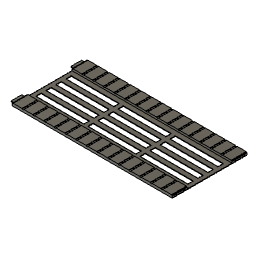
Banc de test linéaire part 2 (Autodesk Fusion 360 design; units mm, degrees)
Autodesk Fusion 360 part; units mm, degrees
sketch "Esquisse1" plane through (0, 0, 0) normal (0, 0, 1) x (1, 0, 0)
  line L0 (0, 0) -> (150, 0)
  line L1 (150, 0) -> (150, 70)
  line L2 (150, 70) -> (0, 70)
  line L3 (0, 70) -> (0, 0)
  dimension "d1" = 70
  dimension "d2" = 150
  constraint horizontal L0
  constraint vertical L1
  constraint horizontal L2
  constraint vertical L3
  constraint coincident L0.start L3.end
  measures "d1" distance of L0.start L2.end
  measures "d2" distance of L0.start L0.end
extrude "Extrusion1" add sketch "Esquisse1" along normal blind 2.5
sketch "Esquisse2" plane through (0, 0, 2.5) normal (0, 0, 1) x (-1, 0, 0)
  line L0 (0, -70) -> (0, 0)
  line L1 (0, 0) -> (-150, 0)
  line L2 (-150, 0) -> (-150, -70)
  line L3 (-150, -70) -> (0, -70)
  line L4 (0, -70) -> (-150, 0) construction
  line L5 (-150, -70) -> (0, 0) construction
  line L6 (0, -14) -> (-150, -14)
  line L7 (-150, -14) -> (-150, -56)
  line L8 (-150, -56) -> (0, -56)
  line L9 (0, -56) -> (0, -14)
  line L10 (0, -14) -> (-150, -56) construction
  line L11 (-150, -14) -> (0, -56) construction
  point P0 (-75, -35)
  dimension "d5" = 42
  dimension "d8" = 150
  constraint coincident L0.start L3.end
  constraint coincident L1.end L2.start
  constraint coincident L2.end L3.start
  constraint coincident L0.end L1.start
  constraint horizontal L6
  constraint perpendicular L6 L7
  constraint parallel L6 L8
  constraint parallel L7 L9
  constraint coincident L10 P0
  constraint coincident L11 P0
  constraint midpoint L4 P0
  measures "d5" distance of L6.end L7.end
  measures "d8" distance of L6.start L6.end
extrude "Extrusion2" cut sketch "Esquisse2" against normal blind 2 contours L0 L2 L6 L7 L8 L9
sketch "Esquisse3" plane through (0, 0, 2.5) normal (0, 0, 1) x (-1, 0, 0)
  line L0 (-150, -14) -> (0, -14)
  line L1 (0, -14) -> (0, 0)
  line L2 (0, 0) -> (-150, 0)
  line L3 (-150, 0) -> (-150, -14)
  line L4 (-0.75, 0) -> (0.75, 0)
  line L5 (0.75, 0) -> (0.75, -14)
  line L6 (0.75, -14) -> (-0.75, -14)
  line L7 (-0.75, -14) -> (-0.75, 0)
  line L8 (-10.75, -14) -> (-10.75, 0)
  line L9 (-9.25, -14) -> (-10.75, -14)
  line L10 (-9.25, 0) -> (-9.25, -14)
  line L11 (-10.75, 0) -> (-9.25, 0)
  line L12 (-19.25, 0) -> (-19.25, -14)
  line L13 (-20.75, -14) -> (-20.75, 0)
  line L14 (-19.25, -14) -> (-20.75, -14)
  line L15 (-20.75, 0) -> (-19.25, 0)
  line L16 (-29.25, 0) -> (-29.25, -14)
  line L17 (-29.25, -14) -> (-30.75, -14)
  line L18 (-30.75, -14) -> (-30.75, 0)
  line L19 (-30.75, 0) -> (-29.25, 0)
  line L20 (-40.75, -14) -> (-40.75, 0)
  line L21 (-39.25, -14) -> (-40.75, -14)
  line L22 (-39.25, 0) -> (-39.25, -14)
  line L23 (-40.75, 0) -> (-39.25, 0)
  line L24 (-50.75, -14) -> (-50.75, 0)
  line L25 (-49.25, -14) -> (-50.75, -14)
  line L26 (-49.25, 0) -> (-49.25, -14)
  line L27 (-50.75, 0) -> (-49.25, 0)
  line L28 (-59.25, -14) -> (-60.75, -14)
  line L29 (-60.75, -14) -> (-60.75, 0)
  line L30 (-59.25, 0) -> (-59.25, -14)
  line L31 (-60.75, 0) -> (-59.25, 0)
  line L32 (-69.25, 0) -> (-69.25, -14)
  line L33 (-69.25, -14) -> (-70.75, -14)
  line L34 (-70.75, -14) -> (-70.75, 0)
  line L35 (-70.75, 0) -> (-69.25, 0)
  line L36 (-79.25, 0) -> (-79.25, -14)
  line L37 (-79.25, -14) -> (-80.75, -14)
  line L38 (-80.75, -14) -> (-80.75, 0)
  line L39 (-80.75, 0) -> (-79.25, 0)
  line L40 (-90.75, -14) -> (-90.75, 0)
  line L41 (-89.25, -14) -> (-90.75, -14)
  line L42 (-89.25, 0) -> (-89.25, -14)
  line L43 (-90.75, 0) -> (-89.25, 0)
  line L44 (-99.25, -14) -> (-100.75, -14)
  line L45 (-100.75, -14) -> (-100.75, 0)
  line L46 (-99.25, 0) -> (-99.25, -14)
  line L47 (-100.75, 0) -> (-99.25, 0)
  line L48 (-109.25, 0) -> (-109.25, -14)
  line L49 (-109.25, -14) -> (-110.75, -14)
  line L50 (-110.75, -14) -> (-110.75, 0)
  line L51 (-110.75, 0) -> (-109.25, 0)
  line L52 (-119.25, -14) -> (-120.75, -14)
  line L53 (-120.75, -14) -> (-120.75, 0)
  line L54 (-119.25, 0) -> (-119.25, -14)
  line L55 (-120.75, 0) -> (-119.25, 0)
  line L56 (-129.25, -14) -> (-130.75, -14)
  line L57 (-130.75, -14) -> (-130.75, 0)
  line L58 (-129.25, 0) -> (-129.25, -14)
  line L59 (-130.75, 0) -> (-129.25, 0)
  line L60 (-150.75, -14) -> (-150.75, 0)
  line L61 (-149.25, -14) -> (-150.75, -14)
  line L62 (-149.25, 0) -> (-149.25, -14)
  line L63 (-150.75, 0) -> (-149.25, 0)
  line L64 (-139.25, -14) -> (-140.75, -14)
  line L65 (-140.75, -14) -> (-140.75, 0)
  line L66 (-140.75, 0) -> (-139.25, 0)
  line L67 (-139.25, 0) -> (-139.25, -14)
  line L68 (-80.75, -56) -> (-79.25, -56)
  line L69 (-70.75, -56) -> (-69.25, -56)
  line L70 (-89.25, -56) -> (-89.25, -70)
  line L71 (-60.75, -70) -> (-60.75, -56)
  line L72 (-39.25, -70) -> (-40.75, -70)
  line L73 (-29.25, -70) -> (-30.75, -70)
  line L74 (-129.25, -70) -> (-130.75, -70)
  line L75 (-110.75, -56) -> (-109.25, -56)
  line L76 (-20.75, -56) -> (-19.25, -56)
  line L77 (-69.25, -56) -> (-69.25, -70)
  line L78 (0.75, -70) -> (-0.75, -70)
  line L79 (-99.25, -70) -> (-100.75, -70)
  line L80 (-59.25, -70) -> (-60.75, -70)
  line L81 (-10.75, -70) -> (-10.75, -56)
  line L82 (-49.25, -56) -> (-49.25, -70)
  line L83 (-10.75, -56) -> (-9.25, -56)
  line L84 (-140.75, -56) -> (-139.25, -56)
  line L85 (-130.75, -56) -> (-129.25, -56)
  line L86 (-140.75, -70) -> (-140.75, -56)
  line L87 (-149.25, -56) -> (-149.25, -70)
  line L88 (-119.25, -56) -> (-119.25, -70)
  line L89 (-99.25, -56) -> (-99.25, -70)
  line L90 (-9.25, -56) -> (-9.25, -70)
  line L91 (-50.75, -56) -> (-49.25, -56)
  line L92 (-100.75, -70) -> (-100.75, -56)
  line L93 (-59.25, -56) -> (-59.25, -70)
  line L94 (-130.75, -70) -> (-130.75, -56)
  line L95 (-40.75, -70) -> (-40.75, -56)
  line L96 (-9.25, -70) -> (-10.75, -70)
  line L97 (-30.75, -56) -> (-29.25, -56)
  line L98 (-19.25, -70) -> (-20.75, -70)
  line L99 (-19.25, -56) -> (-19.25, -70)
  line L100 (-109.25, -56) -> (-109.25, -70)
  line L101 (-129.25, -56) -> (-129.25, -70)
  line L102 (-0.75, -70) -> (-0.75, -56)
  line L103 (-70.75, -70) -> (-70.75, -56)
  line L104 (-79.25, -56) -> (-79.25, -70)
  line L105 (-49.25, -70) -> (-50.75, -70)
  line L106 (-80.75, -70) -> (-80.75, -56)
  line L107 (-109.25, -70) -> (-110.75, -70)
  line L108 (-39.25, -56) -> (-39.25, -70)
  line L109 (-139.25, -70) -> (-140.75, -70)
  line L110 (-30.75, -70) -> (-30.75, -56)
  line L111 (-29.25, -56) -> (-29.25, -70)
  line L112 (-100.75, -56) -> (-99.25, -56)
  line L113 (-150.75, -70) -> (-150.75, -56)
  line L114 (-119.25, -70) -> (-120.75, -70)
  line L115 (-139.25, -56) -> (-139.25, -70)
  line L116 (-120.75, -70) -> (-120.75, -56)
  line L117 (-150.75, -56) -> (-149.25, -56)
  line L118 (-149.25, -70) -> (-150.75, -70)
  line L119 (-69.25, -70) -> (-70.75, -70)
  line L120 (-0.75, -56) -> (0.75, -56)
  line L121 (-120.75, -56) -> (-119.25, -56)
  line L122 (0.75, -56) -> (0.75, -70)
  line L123 (-110.75, -70) -> (-110.75, -56)
  line L124 (-40.75, -56) -> (-39.25, -56)
  line L125 (-90.75, -56) -> (-89.25, -56)
  line L126 (-50.75, -70) -> (-50.75, -56)
  line L127 (-89.25, -70) -> (-90.75, -70)
  line L128 (-90.75, -70) -> (-90.75, -56)
  line L129 (-79.25, -70) -> (-80.75, -70)
  line L130 (-20.75, -70) -> (-20.75, -56)
  line L131 (-60.75, -56) -> (-59.25, -56)
  dimension "d9" = 1.5
  dimension "d10" = 0.75
  dimension "d11" = 1.5
  dimension "d12" = 1.5
  dimension "d13" = 1.5
  dimension "d14" = 1.5
  dimension "d15" = 1.5
  dimension "d16" = 1.5
  dimension "d17" = 1.5
  dimension "d18" = 1.5
  dimension "d19" = 1.5
  dimension "d20" = 1.5
  dimension "d21" = 1.5
  dimension "d22" = 1.5
  dimension "d23" = 1.5
  dimension "d24" = 1.5
  dimension "d25" = 1.5
  dimension "d26" = 1.5
  dimension "d27" = 1.5
  dimension "d28" = 1.5
  dimension "d29" = 1.5
  dimension "d30" = 1.5
  dimension "d31" = 1.5
  dimension "d32" = 1.5
  dimension "d33" = 1.5
  dimension "d34" = 1.5
  dimension "d35" = 1.5
  dimension "d36" = 1.5
  dimension "d37" = 1.5
  dimension "d38" = 1.5
  dimension "d39" = 1.5
  dimension "d40" = 1.5
  dimension "d41" = 1.5
  constraint horizontal L4
  constraint vertical L5
  constraint horizontal L6
  constraint vertical L7
  constraint coincident L2 L4.start
  constraint horizontal L11
  constraint vertical L10
  constraint horizontal L9
  constraint vertical L8
  constraint horizontal L15
  constraint vertical L12
  constraint horizontal L14
  constraint vertical L13
  constraint horizontal L19
  constraint vertical L16
  constraint horizontal L17
  constraint vertical L18
  constraint horizontal L23
  constraint vertical L22
  constraint horizontal L21
  constraint vertical L20
  constraint horizontal L27
  constraint vertical L26
  constraint horizontal L25
  constraint vertical L24
  constraint horizontal L31
  constraint vertical L30
  constraint horizontal L28
  constraint vertical L29
  constraint horizontal L35
  constraint vertical L32
  constraint horizontal L33
  constraint vertical L34
  constraint horizontal L39
  constraint vertical L36
  constraint horizontal L37
  constraint vertical L38
  constraint horizontal L43
  constraint vertical L42
  constraint horizontal L41
  constraint vertical L40
  constraint horizontal L47
  constraint vertical L46
  constraint horizontal L44
  constraint vertical L45
  constraint horizontal L51
  constraint vertical L48
  constraint horizontal L49
  constraint vertical L50
  constraint horizontal L55
  constraint vertical L54
  constraint horizontal L52
  constraint vertical L53
  constraint horizontal L59
  constraint vertical L58
  constraint horizontal L56
  constraint vertical L57
  constraint horizontal L66
  constraint vertical L67
  constraint horizontal L64
  constraint vertical L65
  constraint horizontal L63
  constraint vertical L62
  constraint horizontal L61
  constraint vertical L60
  constraint horizontal L120
  constraint vertical L122
  constraint horizontal L78
  constraint vertical L102
  constraint horizontal L83
  constraint vertical L90
  constraint horizontal L96
  constraint vertical L81
  constraint horizontal L76
  constraint vertical L99
  constraint horizontal L98
  constraint vertical L130
  constraint horizontal L97
  constraint vertical L111
  constraint horizontal L73
  constraint vertical L110
  constraint horizontal L124
  constraint vertical L108
  constraint horizontal L72
  constraint vertical L95
  constraint horizontal L91
  constraint vertical L82
  constraint horizontal L105
  constraint vertical L126
  constraint horizontal L131
  constraint vertical L93
  constraint horizontal L80
  constraint vertical L71
  constraint horizontal L69
  constraint vertical L77
  constraint horizontal L119
  constraint vertical L103
  constraint horizontal L68
  constraint vertical L104
  constraint horizontal L129
  constraint vertical L106
  constraint horizontal L125
  constraint vertical L70
  constraint horizontal L127
  constraint vertical L128
  constraint horizontal L112
  constraint vertical L89
  constraint horizontal L79
  constraint vertical L92
  constraint horizontal L75
  constraint vertical L100
  constraint horizontal L107
  constraint vertical L123
  constraint horizontal L121
  constraint vertical L88
  constraint horizontal L114
  constraint vertical L116
  constraint horizontal L85
  constraint vertical L101
  constraint horizontal L74
  constraint vertical L94
  constraint horizontal L84
  constraint vertical L115
  constraint horizontal L109
  constraint vertical L86
  constraint horizontal L117
  constraint vertical L87
  constraint horizontal L118
  constraint vertical L113
  measures "d9" distance of L5.end L6.end
  measures "d10" distance of L1 L7
  measures "d11" distance of L9.start L8.start
  measures "d12" distance of L12.end L13.start
  measures "d13" distance of L17.end L16.end
  measures "d14" distance of L20.start L21.start
  measures "d15" distance of L25.start L24.start
  measures "d16" distance of L28.start L28.end
  measures "d17" distance of L33.end L32.end
  measures "d18" distance of L37.end L36.end
  measures "d19" distance of L40.start L41.start
  measures "d20" distance of L44.start L44.end
  measures "d21" distance of L48.end L49.end
  measures "d22" distance of L52.start L52.end
  measures "d23" distance of L56.end L56.start
  measures "d24" distance of L64.end L64.start
  measures "d25" distance of L61.start L60.start
  measures "d26" distance of L78.start L78.end
  measures "d27" distance of L90.end L81.start
  measures "d28" distance of L98.end L98.start
  measures "d29" distance of L73.end L73.start
  measures "d30" distance of L72.start L72.end
  measures "d31" distance of L82.end L105.end
  measures "d32" distance of L71.start L80.start
  measures "d33" distance of L103.start L77.end
  measures "d34" distance of L106.start L104.end
  measures "d35" distance of L70.end L127.end
  measures "d36" distance of L79.start L79.end
  measures "d37" distance of L100.end L107.end
  measures "d38" distance of L114.end L88.end
  measures "d39" distance of L74.start L74.end
  measures "d40" distance of L86.start L109.start
  measures "d41" distance of L113.start L87.end
extrude "Extrusion3" cut sketch "Esquisse3" against normal blind 0.4 contours L0 L2 L3 L61 L62 L63 | L3 L60 L61 L63 | L0 L2 L64 L65 L66 L67 | L0 L2 L56 L57 L58 L59 | L0 L2 L52 L53 L54 L55 | L0 L2 L48 L49 L50 L51 | L0 L2 L44 L45 L46 L47 | L0 L2 L40 L41 L42 L43 | L0 L2 L36 L37 L38 L39 | L0 L2 L32 L33 L34 L35 | L0 L2 L28 L29 L30 L31 | L0 L2 L24 L25 L26 L27 | L0 L2 L20 L21 L22 L23 | L0 L2 L16 L17 L18 L19 | L0 L2 L12 L13 L14 L15 | L0 L2 L8 L9 L10 L11 | L0 L1 L2 L4 L6 L7 | L1 L4 L5 L6 | L68 L104 L106 L129 | L69 L77 L103 L119 | L70 L125 L127 L128 | L71 L80 L93 L131 | L72 L95 L108 L124 | L73 L97 L110 L111 | L74 L85 L94 L101 | L75 L100 L107 L123 | L76 L98 L99 L130 | L78 L102 L120 L122 | L79 L89 L92 L112 | L81 L83 L90 L96 | L82 L91 L105 L126 | L84 L86 L109 L115 | L87 L113 L117 L118 | L88 L114 L116 L121
sketch "Esquisse4" plane through (0, 0, 0.5) normal (0, 0, 1) x (-1, 0, 0)
  line L0 (0, -56) -> (0, -14)
  line L1 (0, -14) -> (-150, -14)
  line L2 (-150, -14) -> (-150, -56)
  line L3 (-150, -56) -> (0, -56)
  line L4 (-3.75, -51.6) -> (-48.75, -51.6)
  line L5 (-48.75, -51.6) -> (-48.75, -46.6)
  line L6 (-48.75, -46.6) -> (-3.75, -46.6)
  line L7 (-3.75, -46.6) -> (-3.75, -51.6)
  line L8 (-48.75, -37.2) -> (-3.75, -37.2)
  line L9 (-3.75, -42.2) -> (-48.75, -42.2)
  line L10 (-48.75, -42.2) -> (-48.75, -37.2)
  line L11 (-3.75, -37.2) -> (-3.75, -42.2)
  line L12 (-3.75, -27.8) -> (-3.75, -32.8)
  line L13 (-48.75, -27.8) -> (-3.75, -27.8)
  line L14 (-48.75, -23.4) -> (-48.75, -18.4)
  line L15 (-48.75, -18.4) -> (-3.75, -18.4)
  line L16 (-3.75, -23.4) -> (-48.75, -23.4)
  line L17 (-48.75, -32.8) -> (-48.75, -27.8)
  line L18 (-3.75, -18.4) -> (-3.75, -23.4)
  line L19 (-3.75, -32.8) -> (-48.75, -32.8)
  line L20 (-52.5, -51.6) -> (-97.5, -51.6)
  line L21 (-97.5, -18.4) -> (-52.5, -18.4)
  line L22 (-97.5, -51.6) -> (-97.5, -46.6)
  line L23 (-97.5, -42.2) -> (-97.5, -37.2)
  line L24 (-97.5, -23.4) -> (-97.5, -18.4)
  line L25 (-52.5, -32.8) -> (-97.5, -32.8)
  line L26 (-97.5, -27.8) -> (-52.5, -27.8)
  line L27 (-97.5, -46.6) -> (-52.5, -46.6)
  line L28 (-52.5, -37.2) -> (-52.5, -42.2)
  line L29 (-52.5, -23.4) -> (-97.5, -23.4)
  line L30 (-97.5, -37.2) -> (-52.5, -37.2)
  line L31 (-52.5, -42.2) -> (-97.5, -42.2)
  line L32 (-52.5, -46.6) -> (-52.5, -51.6)
  line L33 (-97.5, -32.8) -> (-97.5, -27.8)
  line L34 (-52.5, -18.4) -> (-52.5, -23.4)
  line L35 (-52.5, -27.8) -> (-52.5, -32.8)
  line L36 (-101.25, -37.2) -> (-101.25, -42.2)
  line L37 (-146.25, -51.6) -> (-146.25, -46.6)
  line L38 (-101.25, -46.6) -> (-101.25, -51.6)
  line L39 (-101.25, -32.8) -> (-146.25, -32.8)
  line L40 (-146.25, -27.8) -> (-101.25, -27.8)
  line L41 (-101.25, -42.2) -> (-146.25, -42.2)
  line L42 (-146.25, -37.2) -> (-101.25, -37.2)
  line L43 (-146.25, -23.4) -> (-146.25, -18.4)
  line L44 (-101.25, -23.4) -> (-146.25, -23.4)
  line L45 (-101.25, -51.6) -> (-146.25, -51.6)
  line L46 (-146.25, -46.6) -> (-101.25, -46.6)
  line L47 (-146.25, -32.8) -> (-146.25, -27.8)
  line L48 (-146.25, -18.4) -> (-101.25, -18.4)
  line L49 (-146.25, -42.2) -> (-146.25, -37.2)
  line L50 (-101.25, -18.4) -> (-101.25, -23.4)
  line L51 (-101.25, -27.8) -> (-101.25, -32.8)
  dimension "d44" = 4.4
  dimension "d45" = 4.4
  dimension "d46" = 4.4
  dimension "d47" = 4.4
  dimension "d48" = 4.4
  dimension "d49" = 4.4
  dimension "d50" = 4.4
  constraint horizontal L4
  constraint vertical L5
  constraint horizontal L6
  constraint vertical L7
  constraint horizontal L9
  constraint vertical L10
  constraint horizontal L8
  constraint vertical L11
  constraint horizontal L19
  constraint vertical L17
  constraint horizontal L13
  constraint vertical L12
  constraint horizontal L16
  constraint vertical L14
  constraint horizontal L15
  constraint vertical L18
  constraint horizontal L20
  constraint vertical L22
  constraint horizontal L27
  constraint vertical L32
  constraint horizontal L31
  constraint vertical L23
  constraint horizontal L30
  constraint vertical L28
  constraint horizontal L25
  constraint vertical L33
  constraint horizontal L26
  constraint vertical L35
  constraint horizontal L29
  constraint vertical L24
  constraint horizontal L21
  constraint vertical L34
  constraint horizontal L45
  constraint vertical L37
  constraint horizontal L46
  constraint vertical L38
  constraint horizontal L41
  constraint vertical L49
  constraint horizontal L42
  constraint vertical L36
  constraint horizontal L39
  constraint vertical L47
  constraint horizontal L40
  constraint vertical L51
  constraint horizontal L44
  constraint vertical L43
  constraint horizontal L48
  constraint vertical L50
  measures "d44" distance of L3 L4
  measures "d45" distance of L6 L9
  measures "d46" distance of L13 L16
  measures "d47" distance of L27 L31
  measures "d48" distance of L26 L29
  measures "d49" distance of L41 L46
  measures "d50" distance of L40 L44
extrude "Extrusion4" cut sketch "Esquisse4" against normal blind 5 contours L4 L5 L6 L7 | L8 L9 L10 L11 | L12 L13 L17 L19 | L14 L15 L16 L18 | L20 L22 L27 L32 | L21 L24 L29 L34 | L23 L28 L30 L31 | L25 L26 L33 L35 | L36 L41 L42 L49 | L37 L38 L45 L46 | L39 L40 L47 L51 | L43 L44 L48 L50
sketch "Esquisse5" plane through (0, 0, 0) normal (-1, 0, 0) x (0, -1, 0)
  line L0 (-56, 2.1) -> (-70, 2.1)
  line L1 (-70, 2.1) -> (-70, 0)
  line L2 (-70, 0) -> (0, 0)
  line L3 (0, 0) -> (0, 2.1)
  line L4 (0, 2.1) -> (-14, 2.1)
  line L5 (-14, 2.1) -> (-14, 0.5)
  line L6 (-14, 0.5) -> (-56, 0.5)
  line L7 (-56, 0.5) -> (-56, 2.1)
  line L8 (-68, 1.55) -> (-58, 1.55)
  line L9 (-58, 1.55) -> (-58, 0.55)
  line L10 (-58, 0.55) -> (-68, 0.55)
  line L11 (-68, 0.55) -> (-68, 1.55)
  line L12 (-68, 1.55) -> (-58, 0.55) construction
  line L13 (-58, 1.55) -> (-68, 0.55) construction
  line L14 (0, 2.1) -> (-14, 0) construction
  line L15 (-14, 2.1) -> (0, 0) construction
  line L16 (-12, 0.55) -> (-2, 0.55)
  line L17 (-2, 0.55) -> (-2, 1.55)
  line L18 (-2, 1.55) -> (-12, 1.55)
  line L19 (-12, 1.55) -> (-12, 0.55)
  line L20 (-12, 0.55) -> (-2, 1.55) construction
  line L21 (-2, 0.55) -> (-12, 1.55) construction
  point P0 (-63, 1.05)
  point P1 (-7, 1.05)
  dimension "d53" = 10
  dimension "d54" = 1
  dimension "d55" = 10
  dimension "d56" = 1
  constraint horizontal L8
  constraint perpendicular L8 L9
  constraint parallel L8 L10
  constraint parallel L9 L11
  constraint coincident L12 P0
  constraint coincident L13 P0
  constraint coincident L3.end L4.start
  constraint coincident L2 L14.end
  constraint coincident L4.end L5.start
  constraint coincident L2.end L3.start
  constraint horizontal L16
  constraint perpendicular L16 L17
  constraint parallel L16 L18
  constraint parallel L17 L19
  constraint coincident L20 P1
  constraint coincident L21 P1
  constraint midpoint L14 P1
  measures "d53" distance of L9.end L10.end
  measures "d54" distance of L8.end L9.end
  measures "d55" distance of L17.end L18.end
  measures "d56" distance of L16.end L17.end
extrude "Extrusion5" add sketch "Esquisse5" along normal blind 3 contours L8 L9 L10 L11 | L16 L17 L18 L19
sketch "Esquisse6" plane through (150, 0, 0) normal (1, 0, 0) x (0, 1, 0)
  line L0 (14, 2.1) -> (0, 2.1)
  line L1 (0, 2.1) -> (0, 0)
  line L2 (0, 0) -> (70, 0)
  line L3 (70, 0) -> (70, 2.1)
  line L4 (70, 2.1) -> (56, 2.1)
  line L5 (56, 2.1) -> (56, 0.5)
  line L6 (56, 0.5) -> (14, 0.5)
  line L7 (14, 0.5) -> (14, 2.1)
  line L8 (1.9, 0.45) -> (12.1, 0.45)
  line L9 (12.1, 0.45) -> (12.1, 1.65)
  line L10 (12.1, 1.65) -> (1.9, 1.65)
  line L11 (1.9, 1.65) -> (1.9, 0.45)
  line L12 (1.9, 0.45) -> (12.1, 1.65) construction
  line L13 (12.1, 0.45) -> (1.9, 1.65) construction
  line L14 (70, 2.1) -> (56, 0) construction
  line L15 (56, 2.1) -> (70, 0) construction
  line L16 (57.9, 0.45) -> (68.1, 0.45)
  line L17 (68.1, 0.45) -> (68.1, 1.65)
  line L18 (68.1, 1.65) -> (57.9, 1.65)
  line L19 (57.9, 1.65) -> (57.9, 0.45)
  line L20 (57.9, 0.45) -> (68.1, 1.65) construction
  line L21 (68.1, 0.45) -> (57.9, 1.65) construction
  point P0 (7, 1.05)
  point P1 (63, 1.05)
  dimension "d59" = 10.2
  dimension "d60" = 1.2
  dimension "d61" = 10.2
  dimension "d62" = 1.2
  constraint horizontal L8
  constraint perpendicular L8 L9
  constraint parallel L8 L10
  constraint parallel L9 L11
  constraint coincident L12 P0
  constraint coincident L13 P0
  constraint coincident L3.end L4.start
  constraint coincident L2 L14.end
  constraint coincident L4.end L5.start
  constraint coincident L2.end L3.start
  constraint horizontal L16
  constraint perpendicular L16 L17
  constraint parallel L16 L18
  constraint parallel L17 L19
  constraint coincident L20 P1
  constraint coincident L21 P1
  constraint midpoint L15 P1
  measures "d59" distance of L9.end L10.end
  measures "d60" distance of L8.end L9.end
  measures "d61" distance of L17.end L18.end
  measures "d62" distance of L16.end L17.end
extrude "Extrusion6" cut sketch "Esquisse6" against normal blind 3.5 contours L8 L9 L10 L11 | L16 L17 L18 L19
